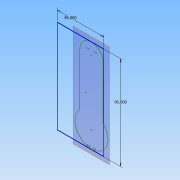
# Autodesk Inventor part: Ply Leftover stock
Saved by Autodesk Inventor 2013 (Build 170138000, 138)
## iProperties
Created: 2018-08-03
Part Number: Ply Leftover stock
Material: Generic
Document SubType Name: Modeling
Designer: Jeff Vyduna
Density: 1 g/cm^3
Author: Jeff Vyduna
Autodesk Inventor part; units mm, degrees
ref_plane "YZ Plane" through (0, 0, 0) normal (1, 0, 0) x (0, 1, 0)
ref_plane "XZ Plane" through (0, 0, 0) normal (0, 1, 0) x (-1, 0, 0)
ref_plane "XY Plane" through (0, 0, 0) normal (0, 0, 1) x (1, 0, 0)
ref_plane "Work Plane1" through (0, 0, -18.034) normal (0, 0, -1) x (-1, 0, 0)
sketch "Sketch1" plane through (0, 0, -18.034) normal (0, 0, -1) x (-1, 0, 0)
  line L0 (-579.8602, -1225.5472) -> (639.3398, -1225.5472)
  line L1 (639.3398, -1225.5472) -> (639.3398, 1212.8528)
  line L2 (639.3398, 1212.8528) -> (-579.8602, 1212.8528)
  line L3 (-579.8602, 1212.8528) -> (-579.8602, -1225.5472)
  circle A0 centre (-78.2102, 1018.4732) radius 9.525 projected
  circle A1 centre (-217.9102, 1018.4732) radius 9.525 projected
  circle A2 centre (-51.2227, -1165.9268) radius 9.525 projected
  circle A3 centre (-244.8977, -1165.9268) radius 9.525 projected
  circle A4 centre (-97.2602, -1165.9268) radius 9.525 projected
  circle A5 centre (-198.8602, -1165.9268) radius 9.525 projected
  circle A6 centre (-263.9477, 1018.4732) radius 9.525 projected
  circle A7 centre (-32.1727, 1018.4732) radius 9.525 projected
  arc A8 (156.7398, 908.0528) -> (-452.8602, 908.0528) centre (-148.0602, 908.0528) ccw projected
  line L4 (-452.8602, 908.0528) -> (-452.8602, -475.1907) projected
  arc A9 (-452.8602, -475.1907) -> (156.7398, -475.1907) centre (-148.0602, -781.0472) ccw projected
  line L5 (156.7398, -475.1907) -> (156.7398, 908.0528) projected
  point P0 (0, 0)
  dimension "d0" = 1219.2
  dimension "d2" = 2438.4
  constraints: 8 end point, 2 parallel, 2 tangent, 1 horizontal, 1 perpendicular
  measures "d0" distance of L1.end L2.end
  measures "d2" distance of L2.end L0.start
extrude "Extrusion1" add sketch "Sketch1" against normal blind 19.05 contours L3 A9 L5 A8 L2 L1 L0 | L3 L2 A8 L4 A9
body "Solid1"
